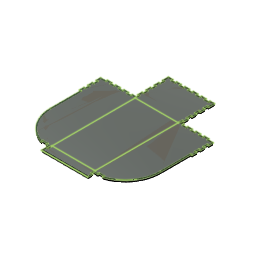
Box (Autodesk Fusion 360 design; units mm, degrees)
Autodesk Fusion 360 part; units mm, degrees
sketch "Sketch1" plane through (0, 0, 0) normal (0, 0, 1) x (1, 0, 0)
  line L0 (0, 0) -> (129.5, 0)
  line L1 (129.5, 0) -> (129.5, 250)
  line L2 (129.5, 250) -> (0, 250)
  line L3 (0, 250) -> (0, 0)
  line L4 (0, 250) -> (0, 350) construction
  line L5 (0, 350) -> (129.5, 350)
  line L6 (129.5, 350) -> (129.5, 250) construction
  line L7 (129.5, 250) -> (233.5, 250) construction
  line L8 (233.5, 250) -> (233.5, 0) construction
  line L9 (233.5, 0) -> (129.5, 0) construction
  line L10 (129.5, 250) -> (129.5, 254)
  line L11 (129.5, 254) -> (142, 254)
  line L12 (142, 254) -> (142, 250)
  line L13 (142, 250) -> (154.5, 250)
  line L14 (154.5, 250) -> (154.5, 254)
  line L15 (154.5, 254) -> (167, 254)
  line L16 (167, 254) -> (167, 250)
  line L17 (167, 250) -> (179.5, 250)
  line L18 (179.5, 250) -> (179.5, 254)
  line L19 (179.5, 254) -> (192, 254)
  line L20 (192, 254) -> (192, 250)
  line L21 (192, 250) -> (204.5, 250)
  line L22 (204.5, 250) -> (204.5, 254)
  line L23 (204.5, 254) -> (217, 254)
  line L24 (217, 254) -> (217, 250)
  line L25 (217, 250) -> (229.5, 250)
  line L26 (229.5, 250) -> (233.5, 250)
  line L27 (233.5, 250) -> (233.5, 237.5)
  line L28 (233.5, 237.5) -> (229.5, 237.5)
  line L29 (229.5, 237.5) -> (229.5, 225)
  line L30 (229.5, 225) -> (233.5, 225)
  line L31 (233.5, 225) -> (233.5, 212.5)
  line L32 (233.5, 212.5) -> (229.5, 212.5)
  line L33 (229.5, 212.5) -> (229.5, 200)
  line L34 (229.5, 200) -> (233.5, 200)
  line L35 (129.5, 250) -> (129.5, 262.5)
  line L36 (129.5, 262.5) -> (133.5, 262.5)
  line L37 (133.5, 262.5) -> (133.5, 275)
  line L38 (133.5, 275) -> (129.5, 275)
  line L39 (129.5, 275) -> (129.5, 287.5)
  line L40 (129.5, 287.5) -> (133.5, 287.5)
  line L41 (133.5, 287.5) -> (133.5, 300)
  line L42 (133.5, 300) -> (129.5, 300)
  line L43 (129.5, 300) -> (129.5, 312.5)
  line L44 (129.5, 312.5) -> (133.5, 312.5)
  line L45 (133.5, 312.5) -> (133.5, 325)
  line L46 (133.5, 325) -> (129.5, 325)
  line L47 (129.5, 325) -> (129.5, 337.5)
  line L48 (129.5, 337.5) -> (133.5, 337.5)
  line L49 (133.5, 337.5) -> (133.5, 350)
  line L50 (129.5, 350) -> (133.5, 350)
  line L51 (129.5, 0) -> (129.5, -25) construction
  line L52 (129.5, -25) -> (0, -25)
  line L53 (0, -25) -> (0, 0) construction
  line L54 (129.5, 0) -> (129.5, -12.5)
  line L55 (129.5, -12.5) -> (133.5, -12.5)
  line L56 (133.5, -12.5) -> (133.5, -25)
  line L57 (129.5, -25) -> (133.5, -25)
  line L58 (129.5, 0) -> (129.5, -4)
  line L59 (129.5, -4) -> (142, -4)
  line L60 (142, -4) -> (142, 0)
  line L61 (142, 0) -> (157.4236, 0)
  line L62 (64.75, 250) -> (64.75, 0) construction
  line L63 (-104, 250) -> (-104, 0) construction
  line L64 (0, -25) -> (-4, -25)
  line L65 (0, 262.5) -> (-4, 262.5)
  line L66 (-4, 300) -> (0, 300)
  line L67 (-4, 325) -> (0, 325)
  line L68 (0, 275) -> (0, 287.5)
  line L69 (0, 337.5) -> (-4, 337.5)
  line L70 (0, 0) -> (0, -12.5)
  line L71 (0, 312.5) -> (-4, 312.5)
  line L72 (-4, 262.5) -> (-4, 275)
  line L73 (-4, 312.5) -> (-4, 325)
  line L74 (-4, 287.5) -> (-4, 300)
  line L75 (-4, 337.5) -> (-4, 350)
  line L76 (0, -12.5) -> (-4, -12.5)
  line L77 (0, 0) -> (0, -4)
  line L78 (-104, 0) -> (0, 0) construction
  line L79 (0, 350) -> (0, 250) construction
  line L80 (0, 300) -> (0, 312.5)
  line L81 (-4, 275) -> (0, 275)
  line L82 (0, 287.5) -> (-4, 287.5)
  line L83 (0, 325) -> (0, 337.5)
  line L84 (0, 250) -> (-104, 250) construction
  line L85 (0, 250) -> (0, 254)
  line L86 (0, 250) -> (0, 262.5)
  line L87 (-4, -12.5) -> (-4, -25)
  line L88 (157.4236, 0) -> (157.4236, -4)
  line L89 (233.5, 200) -> (233.5, 187.5)
  line L90 (233.5, 187.5) -> (229.5, 187.5)
  line L91 (229.5, 187.5) -> (229.5, 96)
  arc A0 (157.4236, -4) -> (229.5, 96) centre (124.091, 96) ccw
  line L92 (133.5, 350) -> (133.5, 354)
  line L93 (133.5, 354) -> (121, 354)
  line L94 (121, 354) -> (121, 350)
  line L95 (121, 350) -> (108.5, 350)
  line L96 (108.5, 350) -> (108.5, 354)
  line L97 (108.5, 354) -> (96, 354)
  line L98 (96, 354) -> (96, 350)
  line L99 (96, 350) -> (83.5, 350)
  line L100 (83.5, 350) -> (83.5, 354)
  line L101 (83.5, 354) -> (71, 354)
  line L102 (71, 354) -> (71, 350)
  line L103 (71, 350) -> (58.5, 350)
  line L104 (58.5, 350) -> (58.5, 354)
  line L105 (58.5, 354) -> (46, 354)
  line L106 (46, 354) -> (46, 350)
  line L107 (46, 350) -> (33.5, 350)
  line L108 (33.5, 350) -> (33.5, 354)
  line L109 (33.5, 354) -> (21, 354)
  line L110 (21, 354) -> (21, 350)
  line L111 (21, 350) -> (8.5, 350)
  line L112 (8.5, 350) -> (8.5, 354)
  line L113 (8.5, 354) -> (-4, 354)
  line L114 (-4, 354) -> (-4, 350)
  line L115 (-100, 250) -> (-104, 250)
  line L116 (-75, 250) -> (-75, 254)
  line L117 (-104, 250) -> (-104, 237.5)
  line L118 (-75, 254) -> (-87.5, 254)
  line L119 (-62.5, 254) -> (-62.5, 250)
  line L120 (-87.5, 254) -> (-87.5, 250)
  line L121 (-12.5, 254) -> (-12.5, 250)
  line L122 (-25, 254) -> (-37.5, 254)
  line L123 (-100, 212.5) -> (-100, 200)
  line L124 (-12.5, 250) -> (-25, 250)
  line L125 (-12.5, -4) -> (-12.5, 0)
  line L126 (-50, 254) -> (-62.5, 254)
  line L127 (-25, 250) -> (-25, 254)
  line L128 (0, 254) -> (-12.5, 254)
  line L129 (-104, 0) -> (0, 0) construction
  line L130 (-62.5, 250) -> (-75, 250)
  line L131 (-37.5, 254) -> (-37.5, 250)
  line L132 (-87.5, 250) -> (-100, 250)
  line L133 (-104, 237.5) -> (-100, 237.5)
  line L134 (-12.5, 0) -> (-27.9236, 0)
  line L135 (-104, 187.5) -> (-100, 187.5)
  line L136 (-100, 187.5) -> (-100, 96)
  line L137 (-27.9236, 0) -> (-27.9236, -4)
  line L138 (-104, 225) -> (-104, 212.5)
  line L139 (-100, 237.5) -> (-100, 225)
  line L140 (-104, 250) -> (-104, 0) construction
  line L141 (-100, 225) -> (-104, 225)
  line L142 (0, -4) -> (-12.5, -4)
  line L143 (-104, 212.5) -> (-100, 212.5)
  arc A1 (-100, 96) -> (-27.9236, -4) centre (5.409, 96) ccw
  line L144 (0, 250) -> (-104, 250) construction
  line L145 (-104, 200) -> (-104, 187.5)
  line L146 (-100, 200) -> (-104, 200)
  line L147 (-50, 250) -> (-50, 254)
  line L148 (-37.5, 250) -> (-50, 250)
  point P0 (233.5, 0)
  point P1 (-104, 0)
  point P2 (-104, 0)
  point P3 (0, 262.5)
  point P4 (-4, 262.5)
  point P5 (0, 250)
  dimension "d85" = 129.5
  dimension "d86" = 250
  dimension "d87" = 100
  dimension "d88" = 129.5
  dimension "d89" = 100
  dimension "d90" = 104
  dimension "d91" = 250
  dimension "d92" = 104
  dimension "d94" = 4
  dimension "d95" = 12.5
  dimension "d96" = 4
  dimension "d97" = 12.5
  dimension "d100" = 25
  dimension "d101" = 0
  dimension "d102" = 12.5
  dimension "d103" = 4
  dimension "d104" = 12.5
  dimension "d105" = 4
  dimension "d106" = 12.5
  dimension "d107" = 4
  dimension "d108" = 12.5
  dimension "d109" = 4
  dimension "d110" = 12.5
  dimension "d111" = 4
  dimension "d112" = 12.5
  dimension "d113" = 4
  dimension "d114" = 12.5
  dimension "d115" = 4
  dimension "d116" = 12.5
  dimension "d117" = 4
  dimension "d118" = 12.5
  dimension "d119" = 4
  dimension "d120" = 12.5
  dimension "d121" = 4
  dimension "d122" = 12.5
  dimension "d123" = 4
  dimension "d124" = 12.5
  dimension "d125" = 25
  dimension "d126" = 129.5
  dimension "d127" = 25
  dimension "d128" = 12.5
  dimension "d129" = 4
  dimension "d130" = 12.5
  dimension "d131" = 4
  dimension "d132" = 4
  dimension "d133" = 12.5
  dimension "d134" = 4
  dimension "d135" = 91.5
  dimension "d141" = 4
  dimension "d144" = 12.5
  dimension "d145" = 4
  dimension "d146" = 91.5
  dimension "d147" = 105.409
  dimension "d148" = 4
  dimension "d149" = 12.5
  dimension "d150" = 4
  dimension "d151" = 12.5
  dimension "d154" = -25
  dimension "d155" = 0
  constraint horizontal L0
  constraint vertical L1
  constraint horizontal L2
  constraint vertical L3
  constraint coincident L0.start L3.end
  constraint perpendicular L2 L4
  constraint perpendicular L4 L5
  constraint perpendicular L2 L6
  constraint perpendicular L1 L7
  constraint perpendicular L7 L8
  constraint perpendicular L1 L9
  constraint perpendicular L2 L10
  constraint perpendicular L6 L11
  constraint perpendicular L11 L12
  constraint perpendicular L12 L13
  constraint perpendicular L26 L27
  constraint perpendicular L27 L28
  constraint perpendicular L28 L29
  constraint perpendicular L8 L30
  constraint perpendicular L30 L31
  constraint perpendicular L31 L32
  constraint perpendicular L32 L33
  constraint perpendicular L33 L34
  constraint perpendicular L11 L35
  constraint perpendicular L35 L36
  constraint perpendicular L36 L37
  constraint perpendicular L6 L38
  constraint perpendicular L38 L39
  constraint perpendicular L39 L40
  constraint perpendicular L40 L41
  constraint perpendicular L6 L42
  constraint perpendicular L42 L43
  constraint perpendicular L43 L44
  constraint perpendicular L44 L45
  constraint perpendicular L45 L46
  constraint perpendicular L44 L47
  constraint perpendicular L47 L48
  constraint perpendicular L48 L49
  constraint perpendicular L9 L51
  constraint perpendicular L51 L52
  constraint perpendicular L0 L53
  constraint perpendicular L9 L54
  constraint perpendicular L51 L55
  constraint perpendicular L55 L56
  constraint perpendicular L56 L57
  constraint perpendicular L9 L58
  constraint perpendicular L54 L59
  constraint perpendicular L9 L60
  constraint coincident L9 P0
  constraint perpendicular L60 L61
  constraint midpoint L2 L62.start
  constraint midpoint L0 L62.end
  constraint symmetric L0.end L62 L0.start
  constraint symmetric L1.end L62 P5
  constraint symmetric L5.end L62 L4.end
  constraint symmetric L7.end L62 L63.start
  constraint symmetric P0 L62 P2
  constraint symmetric L10.end L62 L85.end
  constraint symmetric L35.end L62 P3
  constraint symmetric L36.end L62 P4
  constraint symmetric L37.end L62 L72.end
  constraint symmetric L38.end L62 L68.start
  constraint symmetric L39.end L62 L68.end
  constraint symmetric L40.end L62 L74.start
  constraint symmetric L41.end L62 L66.start
  constraint symmetric L42.end L62 L66.end
  constraint symmetric L43.end L62 L71.start
  constraint symmetric L44.end L62 L71.end
  constraint symmetric L45.end L62 L67.start
  constraint symmetric L46.end L62 L67.end
  constraint symmetric L47.end L62 L69.start
  constraint symmetric L48.end L62 L69.end
  constraint symmetric L49.end L62 L75.end
  constraint symmetric L51.end L62 L52.end
  constraint symmetric L54.end L62 L70.end
  constraint symmetric L55.end L62 L76.end
  constraint symmetric L56.end L62 L64.end
  constraint symmetric L58.end L62 L77.end
  constraint perpendicular L9 L88
  constraint perpendicular L34 L89
  constraint perpendicular L89 L90
  constraint perpendicular L90 L91
  constraint tangent L91 A0
  constraint perpendicular L50 L92
  constraint perpendicular L92 L93
  constraint perpendicular L5 L94
  constraint perpendicular L94 L95
  constraint symmetric L11.end L62 L121.start
  constraint symmetric L12.end L62 L121.end
  constraint symmetric L13.end L62 L124.end
  constraint symmetric L14.end L62 L122.start
  constraint symmetric L15.end L62 L122.end
  constraint symmetric L16.end L62 L131.end
  constraint symmetric L17.end L62 L147.start
  constraint symmetric L18.end L62 L126.start
  constraint symmetric L19.end L62 L119.start
  constraint symmetric L20.end L62 L119.end
  constraint symmetric L21.end L62 L116.start
  constraint symmetric L22.end L62 L116.end
  constraint symmetric L23.end L62 L118.end
  constraint symmetric L24.end L62 L120.end
  constraint symmetric L25.end L62 L115.start
  constraint symmetric L27.end L62 L117.end
  constraint symmetric L28.end L62 L133.end
  constraint symmetric L29.end L62 L139.end
  constraint symmetric L30.end L62 L138.start
  constraint symmetric L31.end L62 L138.end
  constraint symmetric L32.end L62 L123.start
  constraint symmetric L33.end L62 L123.end
  constraint symmetric L34.end L62 L145.start
  constraint symmetric L59.end L62 L125.start
  constraint symmetric L60.end L62 L125.end
  constraint symmetric L61.end L62 L134.end
  constraint symmetric L62 L88.end L137.end
  constraint symmetric L62 L89.end L135.start
  constraint symmetric L62 L90.end L135.end
  constraint symmetric L62 L91.end L136.end
  constraint symmetric L62 A0 A1
  measures "d85" distance of L0.start L0.end
  measures "d86" distance of L0.start P5
  measures "d87" distance of L2.end L4.end
  measures "d88" distance of L4.end L5.end
  measures "d89" distance of L5.end L1.end
  measures "d90" distance of L1.end L7.end
  measures "d91" distance of L7.end P0
  measures "d92" distance of P0 L0.end
  measures "d94" distance of L1.end L10.end
  measures "d95" distance of L10.end L11.end
  measures "d96" distance of L11.end L12.end
  measures "d97" distance of L12.end L13.end
  measures "d102" distance of L7.end L27.end
  measures "d103" distance of L27.end L28.end
  measures "d104" distance of L28.end L29.end
  measures "d105" distance of L29.end L30.end
  measures "d106" distance of L30.end L31.end
  measures "d107" distance of L31.end L32.end
  measures "d108" distance of L32.end L33.end
  measures "d109" distance of L33.end L34.end
  measures "d110" distance of L1.end L35.end
  measures "d111" distance of L35.end L36.end
  measures "d112" distance of L36.end L37.end
  measures "d113" distance of L37.end L38.end
  measures "d114" distance of L38.end L39.end
  measures "d115" distance of L39.end L40.end
  measures "d116" distance of L40.end L41.end
  measures "d117" distance of L41.end L42.end
  measures "d118" distance of L42.end L43.end
  measures "d119" distance of L43.end L44.end
  measures "d120" distance of L44.end L45.end
  measures "d121" distance of L45.end L46.end
  measures "d122" distance of L46.end L47.end
  measures "d123" distance of L47.end L48.end
  measures "d124" distance of L48.end L49.end
  measures "d125" distance of L0.end L51.end
  measures "d126" distance of L51.end L52.end
  measures "d127" distance of L52.end L0.start
  measures "d128" distance of L0.end L54.end
  measures "d129" distance of L54.end L55.end
  measures "d130" distance of L55.end L56.end
  measures "d131" distance of L51.end L56.end
  measures "d132" distance of L0.end L58.end
  measures "d133" distance of L58.end L59.end
  measures "d134" distance of L59.end L60.end
  measures "d135" distance of L60.end P0
  measures "d141" distance of L61.end L88.end
  measures "d144" distance of L34.end L89.end
  measures "d145" distance of L89.end L90.end
  measures "d146" distance of L90.end L91.end
  measures "d147" radius of A0
  measures "d148" distance of L49.end L92.end
  measures "d149" distance of L92.end L93.end
  measures "d150" distance of L93.end L94.end
  measures "d151" distance of L94.end L95.end
extrude "Extrude1" add sketch "Sketch1" along normal blind 5
sketch "Sketch2" plane through (0, 0, 5) normal (0, 0, 1) x (-1, 0, 0)
  line L0 (0, 4) -> (0, 12.5) construction
  line L1 (0, 12.5) -> (4, 12.5) construction
  line L2 (4, 12.5) -> (4, 25) construction
  line L3 (-133.5, 25) -> (-133.5, 12.5) construction
  line L4 (-133.5, 12.5) -> (-129.5, 12.5) construction
  line L5 (-129.5, 12.5) -> (-129.5, 4) construction
  line L6 (-129.5, 4) -> (-142, 4) construction
  line L7 (-142, 4) -> (-142, 0) construction
  line L8 (-142, 0) -> (-157.4236, 0) construction
  line L9 (-233.5, -200) -> (-229.5, -200) construction
  line L10 (-229.5, -200) -> (-229.5, -212.5) construction
  line L11 (-229.5, -212.5) -> (-233.5, -212.5) construction
  line L12 (-233.5, -212.5) -> (-233.5, -225) construction
  line L13 (-233.5, -225) -> (-229.5, -225) construction
  line L14 (-229.5, -225) -> (-229.5, -237.5) construction
  line L15 (-229.5, -237.5) -> (-233.5, -237.5) construction
  line L16 (-233.5, -237.5) -> (-233.5, -250) construction
  line L17 (-233.5, -250) -> (-217, -250) construction
  line L18 (-217, -250) -> (-217, -254) construction
  line L19 (-217, -254) -> (-204.5, -254) construction
  line L20 (-204.5, -254) -> (-204.5, -250) construction
  line L21 (-204.5, -250) -> (-192, -250) construction
  line L22 (-192, -250) -> (-192, -254) construction
  line L23 (-192, -254) -> (-179.5, -254) construction
  line L24 (-179.5, -254) -> (-179.5, -250) construction
  line L25 (-179.5, -250) -> (-167, -250) construction
  line L26 (-167, -250) -> (-167, -254) construction
  line L27 (-167, -254) -> (-154.5, -254) construction
  line L28 (-154.5, -254) -> (-154.5, -250) construction
  line L29 (-154.5, -250) -> (-142, -250) construction
  line L30 (-142, -250) -> (-142, -254) construction
  line L31 (-142, -254) -> (-129.5, -254) construction
  line L32 (-129.5, -254) -> (-129.5, -262.5) construction
  line L33 (-129.5, -262.5) -> (-133.5, -262.5) construction
  line L34 (-133.5, -262.5) -> (-133.5, -275) construction
  line L35 (-133.5, -275) -> (-129.5, -275) construction
  line L36 (-129.5, -275) -> (-129.5, -287.5) construction
  line L37 (-129.5, -287.5) -> (-133.5, -287.5) construction
  line L38 (-133.5, -287.5) -> (-133.5, -300) construction
  line L39 (-133.5, -300) -> (-129.5, -300) construction
  line L40 (-129.5, -300) -> (-129.5, -312.5) construction
  line L41 (-129.5, -312.5) -> (-133.5, -312.5) construction
  line L42 (-133.5, -312.5) -> (-133.5, -325) construction
  line L43 (-133.5, -325) -> (-129.5, -325) construction
  line L44 (-129.5, -325) -> (-129.5, -337.5) construction
  line L45 (-129.5, -337.5) -> (-133.5, -337.5) construction
  line L46 (-133.5, -337.5) -> (-133.5, -354) construction
  line L47 (4, -354) -> (4, -337.5) construction
  line L48 (4, -337.5) -> (0, -337.5) construction
  line L49 (0, -337.5) -> (0, -325) construction
  line L50 (0, -325) -> (4, -325) construction
  line L51 (4, -325) -> (4, -312.5) construction
  line L52 (4, -312.5) -> (0, -312.5) construction
  line L53 (0, -312.5) -> (0, -300) construction
  line L54 (0, -300) -> (4, -300) construction
  line L55 (4, -300) -> (4, -287.5) construction
  line L56 (4, -287.5) -> (0, -287.5) construction
  line L57 (0, -287.5) -> (0, -275) construction
  line L58 (0, -275) -> (4, -275) construction
  line L59 (4, -275) -> (4, -262.5) construction
  line L60 (4, -262.5) -> (0, -262.5) construction
  line L61 (0, -262.5) -> (0, -254) construction
  line L62 (-157.4236, 0) -> (-157.4236, 4)
  arc A0 (-157.4236, 4) -> (-229.5, -96) centre (-124.091, -96) ccw
  line L63 (-229.5, -96) -> (-229.5, -187.5)
  line L64 (-229.5, -187.5) -> (-233.5, -187.5)
  line L65 (-233.5, -187.5) -> (-233.5, -200)
  line L66 (-133.5, -354) -> (-121, -354)
  line L67 (-121, -354) -> (-121, -350)
  line L68 (-121, -350) -> (-108.5, -350)
  line L69 (-108.5, -350) -> (-108.5, -354)
  line L70 (-108.5, -354) -> (-96, -354)
  line L71 (-96, -354) -> (-96, -350)
  line L72 (-96, -350) -> (-83.5, -350)
  line L73 (-83.5, -350) -> (-83.5, -354)
  line L74 (-83.5, -354) -> (-71, -354)
  line L75 (-71, -354) -> (-71, -350)
  line L76 (-71, -350) -> (-58.5, -350)
  line L77 (-58.5, -350) -> (-58.5, -354)
  line L78 (-58.5, -354) -> (-46, -354)
  line L79 (-46, -354) -> (-46, -350)
  line L80 (-46, -350) -> (-33.5, -350)
  line L81 (-33.5, -350) -> (-33.5, -354)
  line L82 (-33.5, -354) -> (-21, -354)
  line L83 (-21, -354) -> (-21, -350)
  line L84 (-21, -350) -> (-8.5, -350)
  line L85 (-8.5, -350) -> (-8.5, -354)
  line L86 (-8.5, -354) -> (4, -354)
  line L87 (0, -254) -> (12.5, -254)
  line L88 (12.5, -254) -> (12.5, -250)
  line L89 (12.5, -250) -> (25, -250)
  line L90 (25, -250) -> (25, -254)
  line L91 (25, -254) -> (37.5, -254)
  line L92 (37.5, -254) -> (37.5, -250)
  line L93 (37.5, -250) -> (50, -250)
  line L94 (50, -250) -> (50, -254)
  line L95 (50, -254) -> (62.5, -254)
  line L96 (62.5, -254) -> (62.5, -250)
  line L97 (62.5, -250) -> (75, -250)
  line L98 (75, -250) -> (75, -254)
  line L99 (75, -254) -> (87.5, -254)
  line L100 (87.5, -254) -> (87.5, -250)
  line L101 (87.5, -250) -> (104, -250)
  line L102 (104, -250) -> (104, -237.5)
  line L103 (104, -237.5) -> (100, -237.5)
  line L104 (100, -237.5) -> (100, -225)
  line L105 (100, -225) -> (104, -225)
  line L106 (104, -225) -> (104, -212.5)
  line L107 (104, -212.5) -> (100, -212.5)
  line L108 (100, -212.5) -> (100, -200)
  line L109 (100, -200) -> (104, -200)
  line L110 (104, -200) -> (104, -187.5)
  line L111 (104, -187.5) -> (100, -187.5)
  line L112 (100, -187.5) -> (100, -96)
  arc A1 (100, -96) -> (27.9236, 4) centre (-5.409, -96) ccw
  line L113 (27.9236, 4) -> (27.9236, 0)
  line L114 (27.9236, 0) -> (12.5, 0)
  line L115 (12.5, 0) -> (12.5, 4)
  line L116 (12.5, 4) -> (0, 4)
  line L117 (-229.8, -200.3) -> (-229.8, -212.2)
  line L118 (-229.8, -212.2) -> (-233.8, -212.2)
  line L119 (-233.8, -212.2) -> (-233.8, -225.3)
  line L120 (-233.8, -225.3) -> (-229.8, -225.3)
  line L121 (-229.8, -225.3) -> (-229.8, -237.2)
  line L122 (-229.8, -237.2) -> (-233.8, -237.2)
  line L123 (-233.8, -237.2) -> (-233.8, -250.3)
  line L124 (-233.8, -250.3) -> (-217.3, -250.3)
  line L125 (-217.3, -250.3) -> (-217.3, -254.3)
  line L126 (-217.3, -254.3) -> (-204.2, -254.3)
  line L127 (-204.2, -254.3) -> (-204.2, -250.3)
  line L128 (-204.2, -250.3) -> (-192.3, -250.3)
  line L129 (-192.3, -250.3) -> (-192.3, -254.3)
  line L130 (-192.3, -254.3) -> (-179.2, -254.3)
  line L131 (-179.2, -254.3) -> (-179.2, -250.3)
  line L132 (-179.2, -250.3) -> (-167.3, -250.3)
  line L133 (-167.3, -250.3) -> (-167.3, -254.3)
  line L134 (-167.3, -254.3) -> (-154.2, -254.3)
  line L135 (-154.2, -254.3) -> (-154.2, -250.3)
  line L136 (-154.2, -250.3) -> (-142.3, -250.3)
  line L137 (-142.3, -250.3) -> (-142.3, -254.3)
  line L138 (-142.3, -254.3) -> (-129.8, -254.3)
  line L139 (-129.8, -254.3) -> (-129.8, -262.2)
  line L140 (-129.8, -262.2) -> (-133.8, -262.2)
  line L141 (-133.8, -262.2) -> (-133.8, -275.3)
  line L142 (-133.8, -275.3) -> (-129.8, -275.3)
  line L143 (-129.8, -275.3) -> (-129.8, -287.2)
  line L144 (-129.8, -287.2) -> (-133.8, -287.2)
  line L145 (-133.8, -287.2) -> (-133.8, -300.3)
  line L146 (-133.8, -300.3) -> (-129.8, -300.3)
  line L147 (-129.8, -300.3) -> (-129.8, -312.2)
  line L148 (-129.8, -312.2) -> (-133.8, -312.2)
  line L149 (-133.8, -312.2) -> (-133.8, -325.3)
  line L150 (-133.8, -325.3) -> (-129.8, -325.3)
  line L151 (-129.8, -325.3) -> (-129.8, -337.2)
  line L152 (-129.8, -337.2) -> (-133.8, -337.2)
  line L153 (-133.8, -337.2) -> (-133.8, -354.3)
  line L154 (-133.8, -354.3) -> (-120.7, -354.3)
  line L155 (-120.7, -354.3) -> (-120.7, -350.3)
  line L156 (-120.7, -350.3) -> (-108.8, -350.3)
  line L157 (-108.8, -350.3) -> (-108.8, -354.3)
  line L158 (-108.8, -354.3) -> (-95.7, -354.3)
  line L159 (-95.7, -354.3) -> (-95.7, -350.3)
  line L160 (-95.7, -350.3) -> (-83.8, -350.3)
  line L161 (-83.8, -350.3) -> (-83.8, -354.3)
  line L162 (-83.8, -354.3) -> (-70.7, -354.3)
  line L163 (-70.7, -354.3) -> (-70.7, -350.3)
  line L164 (-70.7, -350.3) -> (-58.8, -350.3)
  line L165 (-58.8, -350.3) -> (-58.8, -354.3)
  line L166 (-58.8, -354.3) -> (-45.7, -354.3)
  line L167 (-45.7, -354.3) -> (-45.7, -350.3)
  line L168 (-45.7, -350.3) -> (-33.8, -350.3)
  line L169 (-33.8, -350.3) -> (-33.8, -354.3)
  line L170 (-33.8, -354.3) -> (-20.7, -354.3)
  line L171 (-20.7, -354.3) -> (-20.7, -350.3)
  line L172 (-20.7, -350.3) -> (-8.8, -350.3)
  line L173 (-8.8, -350.3) -> (-8.8, -354.3)
  line L174 (-8.8, -354.3) -> (4.3, -354.3)
  line L175 (4.3, -354.3) -> (4.3, -337.2)
  line L176 (4.3, -337.2) -> (0.3, -337.2)
  line L177 (0.3, -337.2) -> (0.3, -325.3)
  line L178 (0.3, -325.3) -> (4.3, -325.3)
  line L179 (4.3, -325.3) -> (4.3, -312.2)
  line L180 (4.3, -312.2) -> (0.3, -312.2)
  line L181 (0.3, -312.2) -> (0.3, -300.3)
  line L182 (0.3, -300.3) -> (4.3, -300.3)
  line L183 (4.3, -300.3) -> (4.3, -287.2)
  line L184 (4.3, -287.2) -> (0.3, -287.2)
  line L185 (0.3, -287.2) -> (0.3, -275.3)
  line L186 (0.3, -275.3) -> (4.3, -275.3)
  line L187 (4.3, -275.3) -> (4.3, -262.2)
  line L188 (4.3, -262.2) -> (0.3, -262.2)
  line L189 (0.3, -262.2) -> (0.3, -254.3)
  line L190 (0.3, -254.3) -> (12.8, -254.3)
  line L191 (12.8, -254.3) -> (12.8, -250.3)
  line L192 (12.8, -250.3) -> (24.7, -250.3)
  line L193 (24.7, -250.3) -> (24.7, -254.3)
  line L194 (24.7, -254.3) -> (37.8, -254.3)
  line L195 (37.8, -254.3) -> (37.8, -250.3)
  line L196 (37.8, -250.3) -> (49.7, -250.3)
  line L197 (49.7, -250.3) -> (49.7, -254.3)
  line L198 (49.7, -254.3) -> (62.8, -254.3)
  line L199 (62.8, -254.3) -> (62.8, -250.3)
  line L200 (62.8, -250.3) -> (74.7, -250.3)
  line L201 (74.7, -250.3) -> (74.7, -254.3)
  line L202 (74.7, -254.3) -> (87.8, -254.3)
  line L203 (87.8, -254.3) -> (87.8, -250.3)
  line L204 (87.8, -250.3) -> (104.3, -250.3)
  line L205 (104.3, -250.3) -> (104.3, -237.2)
  line L206 (104.3, -237.2) -> (100.3, -237.2)
  line L207 (100.3, -237.2) -> (100.3, -225.3)
  line L208 (100.3, -225.3) -> (104.3, -225.3)
  line L209 (104.3, -225.3) -> (104.3, -212.2)
  line L210 (104.3, -212.2) -> (100.3, -212.2)
  line L211 (100.3, -212.2) -> (100.3, -200.3)
  line L212 (100.3, -200.3) -> (104.3, -200.3)
  line L213 (104.3, -200.3) -> (104.3, -187.2)
  line L214 (104.3, -187.2) -> (100.3, -187.2)
  line L215 (100.3, -187.2) -> (100.3, -96)
  arc A2 (100.3, -96) -> (27.6236, 4.4154) centre (-5.409, -96) ccw
  line L216 (27.6236, 4.4154) -> (27.6236, 0.3)
  line L217 (27.6236, 0.3) -> (12.8, 0.3)
  line L218 (12.8, 0.3) -> (12.8, 4.3)
  line L219 (12.8, 4.3) -> (0.3, 4.3)
  line L220 (0.3, 4.3) -> (0.3, 12.2)
  line L221 (0.3, 12.2) -> (4.3, 12.2)
  line L222 (4.3, 12.2) -> (4.3, 27.024)
  line L223 (-133.8, 27.024) -> (-133.8, 12.2)
  line L224 (-133.8, 12.2) -> (-129.8, 12.2)
  line L225 (-129.8, 12.2) -> (-129.8, 4.3)
  line L226 (-129.8, 4.3) -> (-142.3, 4.3)
  line L227 (-142.3, 4.3) -> (-142.3, 0.3)
  line L228 (-142.3, 0.3) -> (-157.1236, 0.3)
  line L229 (-157.1236, 0.3) -> (-157.1236, 4.4154)
  arc A3 (-157.1236, 4.4154) -> (-229.8, -96) centre (-124.091, -96) ccw
  line L230 (-229.8, -96) -> (-229.8, -187.2)
  line L231 (-229.8, -187.2) -> (-233.8, -187.2)
  line L232 (-233.8, -187.2) -> (-233.8, -200.3)
  line L233 (-233.8, -200.3) -> (-229.8, -200.3)
  line L234 (0, 4) -> (0, 0)
  line L235 (0, 0) -> (0, -250)
  line L236 (0, -250) -> (0, -254)
  line L237 (-129.5, -254) -> (-129.5, -250)
  line L238 (-129.5, -250) -> (0, -250)
  line L239 (-129.5, 4) -> (-129.5, 0)
  line L240 (-129.5, 0) -> (0, 0)
  line L241 (-129.5, -250) -> (-129.5, 0)
  line L242 (4.3, 27.024) -> (-133.8, 27.024)
  dimension "d139" = 0.3
  dimension "d212" = 14.824
  dimension "d213" = 14.824
  constraint coincident L0.start L116.end
  constraint coincident L234.end L235.start
  constraint perpendicular L87 L235
  constraint coincident L61.end L87.start
  constraint perpendicular L87 L236
  constraint coincident L31.end L32.start
  constraint perpendicular L31 L237
  constraint perpendicular L236 L238
  constraint coincident L5.end L6.start
  constraint perpendicular L226 L239
  constraint perpendicular L234 L240
  measures "d212" distance of L221.end L222.end
  measures "d213" distance of L223.start L223.end
sketch "Sketch3" plane through (0, 0, 5) normal (0, 0, 1) x (-1, 0, 0)
equation "width = height + 3 * height / ( 2 * number_fingers ) - 2 * Thickness"
equation "length = 250 mm"
equation "height = 100 mm"
equation "Thickness = 4 mm"
equation "number_fingers = 4"
equation "d85 = width"
equation "d86 = length"
equation "d87 = height"
equation "d88 = width"
equation "d89 = height"
equation "d90 = height + Thickness"
equation "d91 = length"
equation "d92 = height + Thickness"
equation "d94 = Thickness"
equation "d95 = height / ( 2 * number_fingers )"
equation "d96 = Thickness"
equation "d97 = height / ( 2 * number_fingers )"
equation "d98 = number_fingers"
equation "d100 = height / number_fingers"
equation "d102 = height / ( 2 * number_fingers )"
equation "d103 = Thickness"
equation "d104 = height / ( 2 * number_fingers )"
equation "d105 = Thickness"
equation "d106 = height / ( 2 * number_fingers )"
equation "d107 = Thickness"
equation "d108 = height / ( 2 * number_fingers )"
equation "d109 = Thickness"
equation "d110 = height / ( 2 * number_fingers )"
equation "d111 = Thickness"
equation "d112 = height / ( 2 * number_fingers )"
equation "d113 = Thickness"
equation "d114 = height / ( 2 * number_fingers )"
equation "d115 = Thickness"
equation "d116 = height / ( 2 * number_fingers )"
equation "d117 = Thickness"
equation "d118 = height / ( 2 * number_fingers )"
equation "d119 = Thickness"
equation "d120 = height / ( 2 * number_fingers )"
equation "d121 = Thickness"
equation "d122 = height / ( 2 * number_fingers )"
equation "d123 = Thickness"
equation "d124 = height / ( 2 * number_fingers )"
equation "d125 = height / number_fingers"
equation "d126 = width"
equation "d127 = height / number_fingers"
equation "d128 = height / ( 2 * number_fingers )"
equation "d129 = Thickness"
equation "d130 = height / ( 2 * number_fingers )"
equation "d131 = Thickness"
equation "d132 = Thickness"
equation "d133 = height / ( 2 * number_fingers )"
equation "d134 = Thickness"
equation "d135 = height + Thickness - height / ( 2 * number_fingers )"
equation "d141 = Thickness"
equation "d144 = height / ( 2 * number_fingers )"
equation "d145 = Thickness"
equation "d146 = length - height * 1.5 / number_fingers - height + Thickness - height / number_fingers"
equation "d148 = Thickness"
equation "d149 = height / ( 2 * number_fingers )"
equation "d150 = Thickness"
equation "d151 = height / ( 2 * number_fingers )"
equation "d154 = height / number_fingers * -1"
equation "d156 = width + 2 * Thickness"
equation "d178 = height / ( 2 * number_fingers )"
equation "d179 = Thickness"
equation "d180 = height / ( 2 * number_fingers )"
equation "d181 = Thickness"
equation "d182 = height / ( 2 * number_fingers )"
equation "d183 = Thickness"
equation "d184 = height / ( 2 * number_fingers )"
equation "d185 = Thickness"
equation "d186 = height"
equation "d187 = height / ( 2 * number_fingers )"
equation "d188 = Thickness"
equation "d189 = height / ( 2 * number_fingers )"
equation "d190 = height / ( 2 * number_fingers )"
equation "d191 = Thickness"
equation "d192 = height / ( 2 * number_fingers )"
equation "d193 = Thickness"
equation "d194 = height / ( 4 * number_fingers )"
equation "d195 = height / ( 2 * number_fingers )"
